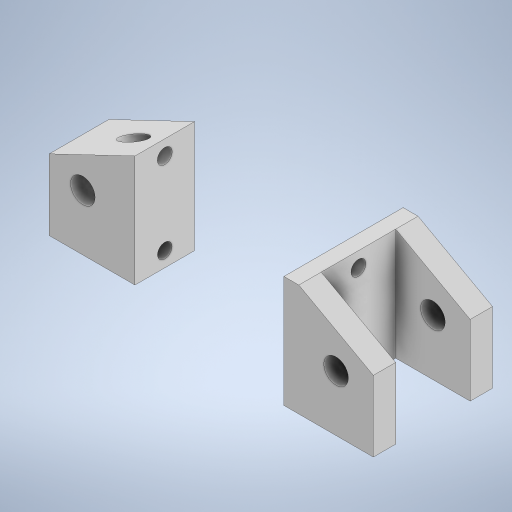
# Autodesk Inventor part: baseFingerLayout
Saved by Autodesk Inventor 2024 (Build 280153000, 153)
## iProperties
Created: 2024-05-29
Part Number: baseFingerLayout
Material: Generic
Document SubType Name: Modeling
Designer: 7008661
Density: 1 g/cm^3
Appearance: Default
Author: 7008661
Autodesk Inventor part; units mm, degrees
ref_plane "YZ Plane" through (0, 0, 0) normal (1, 0, 0) x (0, 1, 0)
ref_plane "XZ Plane" through (0, 0, 0) normal (0, 1, 0) x (-1, 0, 0)
ref_plane "XY Plane" through (0, 0, 0) normal (0, 0, 1) x (1, 0, 0)
sketch "Sketch1" plane through (0, 0, 0) normal (0, 1, 0) x (-1, 0, 0)
  line L0 (-18, -8) -> (18, -8)
  line L1 (18, -8) -> (18, 8)
  line L2 (18, 8) -> (-18, 8)
  line L3 (-18, 8) -> (-18, -8)
  line L4 (-18, -8) -> (18, 8) construction
  line L5 (18, -8) -> (-18, 8) construction
  point P0 (0, 0)
  dimension "d0" = 36
  dimension "d1" = 16
  constraints: 12 end point, 2 midpoint, 2 parallel, 1 horizontal, 1 perpendicular
  measures "d0" distance of L2.end L1.end
  measures "d1" distance of L1.end L0.end
extrude "Extrusion1" add sketch "Sketch1" along normal blind 15
sketch "Sketch2" plane through (18, 0, 8) normal (1, 0, 0) x (0, 0, -1)
  line L0 (16, 15) -> (0, 15) projected
  line L1 (13, 0) -> (3, 0)
  line L2 (3, 0) -> (3, 15)
  line L3 (3, 15) -> (13, 15)
  line L4 (13, 15) -> (13, 0)
  line L5 (13, 0) -> (3, 15) construction
  line L6 (3, 0) -> (13, 15) construction
  point P0 (8, 0)
  point P1 (8, 7.5)
  dimension "d4" = 10
  constraints: 12 end point, 2 midpoint, 2 parallel, 1 horizontal, 1 perpendicular, 1 point on line
  measures "d4" distance of L2.end L3.end
sketch "Sketch3" plane through (-18, 0, 8) normal (0, 0, 1) x (1, 0, 0)
  line L0 (36, 0) -> (36, 15) projected
  line L1 (0, 15) -> (36, 15) projected
  line L2 (36, 0) -> (26, 0)
  line L3 (26, 0) -> (26, 15)
  line L4 (26, 15) -> (36, 15)
  line L5 (36, 15) -> (36, 0)
  circle A0 centre (31, 7.5) radius 1.65
  point P0 (18, 0)
  dimension "d5" = 10
  dimension "d6" = 3.3
  constraints: 8 end point, 2 parallel, 1 centre point, 1 horizontal, 1 perpendicular, 1 point on line
  measures "d5" distance of L3.end L4.end
  measures "d6" diameter of A0
extrude "Extrusion2" cut sketch "Sketch3" against normal blind 21.25 contours A0
chamfer "Chamfer1" distance 10 distance2 5.5 1 edges at (18, 15, 0) measured on face at (17.5, 15, 0)
extrude "Extrusion3" cut sketch "Sketch2" against normal blind 10
sketch "Sketch4" plane through (-18, 0, -8) normal (-1, 0, 0) x (0, 0, 1)
  line L0 (0, 15) -> (16, 15) projected
  line L1 (11.5, 0) -> (4.5, 0)
  line L2 (4.5, 0) -> (4.5, 15)
  line L3 (4.5, 15) -> (11.5, 15)
  line L4 (11.5, 15) -> (11.5, 0)
  line L5 (11.5, 0) -> (4.5, 15) construction
  line L6 (4.5, 0) -> (11.5, 15) construction
  point P0 (8, 0)
  point P1 (8, 7.5)
  dimension "d14" = 7
  constraints: 12 end point, 2 midpoint, 2 parallel, 1 horizontal, 1 perpendicular, 1 point on line
  measures "d14" distance of L2.end L3.end
extrude "Extrusion4" add sketch "Sketch4" along normal blind 11.5
sketch "Sketch5" plane through (-18, 0, 3.5) normal (0, 0, 1) x (1, 0, 0)
  circle A0 centre (-5.75, 7.5) radius 1.65
  point P0 (18, 0)
  dimension "d17" = 3.3
  constraints: 1 centre point
  measures "d17" diameter of A0
extrude "Extrusion5" add sketch "Sketch5" against normal blind 1
chamfer "Chamfer2" distance 6 distance2 11.5 1 edges at (-29.5, 15, 0) measured on face at (-29.5, 14.5, 0)
sketch "Sketch6" plane through (-29.5, 0, -8) normal (-1, 0, 0) x (0, 0, 1)
  point P0 (8, 0)
sketch "Sketch7" plane through (0, 0, 0) normal (0, -1, 0) x (1, 0, 0)
  line L0 (-18, -3.5) -> (-29.5, -3.5) projected
  line L1 (-29.5, 3.5) -> (-18, 3.5) projected
  line L2 (-18, -3.5) -> (-29.5, -3.5)
  line L3 (-29.5, -3.5) -> (-29.5, 3.5)
  line L4 (-29.5, 3.5) -> (-18, 3.5)
  line L5 (-18, 3.5) -> (-18, -3.5)
  point P0 (0, 0)
  constraints: 8 end point, 2 parallel, 1 horizontal, 1 perpendicular
extrude "Extrusion6" add sketch "Sketch7" against normal blind 15
sketch "Sketch8" plane through (-18, 0, -3.5) normal (0, 0, -1) x (-1, 0, 0)
  line L0 (0, 15) -> (11.5, 15) projected
  line L1 (0, 0) -> (11.5, 0) projected
  line L2 (11.5, 15) -> (2.5, 15)
  line L3 (2.5, 15) -> (2.5, 0)
  line L4 (2.5, 0) -> (11.5, 0)
  line L5 (11.5, 0) -> (11.5, 15)
  circle A0 centre (7, 7.5) radius 1.65
  point P0 (-18, 0)
  dimension "d25" = 9
  dimension "d26" = 3.3
  constraints: 8 end point, 2 parallel, 1 centre point, 1 horizontal, 1 perpendicular, 1 point on line
  measures "d25" distance of L4.end L3.end
  measures "d26" diameter of A0
extrude "Extrusion7" cut sketch "Sketch8" along normal mid plane 45.25 contours A0
chamfer "Chamfer3" distance 11.5 distance2 5.5 1 edges at (-29.5, 15, 0) measured on face at (-29, 15, 0)
sketch "Sketch9" plane through (18, 0, -8) normal (0, 0, -1) x (-1, 0, 0)
  point P0 (18, 0)
sketch "Sketch10" plane through (8, 0, 8) normal (1, 0, 0) x (0, 0, -1)
  line L0 (4.5, 15) -> (11.5, 15) projected
  circle A0 centre (8, 13) radius 1
  circle A1 centre (8, 2) radius 0.975
  point P0 (8, 0)
  dimension "d32" = 2
  constraints: 2 centre point
  measures "d32" diameter of A0
extrude "Extrusion8" cut sketch "Sketch10" against normal blind 65.75
sketch "Sketch11" plane through (-29.5, 0, 3.5) normal (0, 0, 1) x (1, 0, 0)
  line L0 (0, 0) -> (0, 9.5) projected
  line L1 (37.5, 15) -> (11.5, 15) projected
  line L2 (0, 9.5) -> (11.5, 15)
  line L3 (47.5, 0) -> (11.5, 0) projected
  line L4 (11.5, 15) -> (11.5, 0)
  line L5 (11.5, 0) -> (0, 0)
  line L6 (0, 0) -> (0, 9.5)
  point P0 (29.5, 0)
  constraints: 8 end point, 3 perpendicular
extrude "Extrusion9" add sketch "Sketch11" along normal blind 0.5
sketch "Sketch12" plane through (-18, 0, -3.5) normal (0, 0, -1) x (-1, 0, 0)
  circle A0 centre (7, 7.5) radius 1.65 projected
  circle A1 centre (7, 7.5) radius 1.65
  point P0 (-18, 0)
  constraints: 1 centre point, 1 coincident
extrude "Extrusion10" cut sketch "Sketch12" against normal blind 9
sketch "Sketch13" plane through (-18, 0, -3.5) normal (0, 0, -1) x (-1, 0, 0)
  point P0 (-18, 0)
sketch "Sketch14" plane through (-18, 0, -3.5) normal (0, 0, -1) x (-1, 0, 0)
  line L0 (0, 0) -> (0, 15) projected
  line L1 (0, 0) -> (0, 15)
  line L2 (11.5, 9.5) -> (11.5, 0) projected
  line L3 (0, 15) -> (11.5, 9.5)
  line L4 (11.5, 9.5) -> (11.5, 0)
  line L5 (11.5, 0) -> (0, 0) projected
  line L6 (11.5, 0) -> (0, 0)
  point P0 (-18, 0)
  constraints: 8 end point, 2 collinear, 1 parallel
extrude "Extrusion11" add sketch "Sketch14" along normal blind 0.5
sketch "Sketch15" plane through (-29.5, 0, 4) normal (0, 0, 1) x (1, 0, 0)
  circle A0 centre (4.5, 7.5) radius 1.65 projected
  circle A1 centre (4.5, 7.5) radius 1.65
  point P0 (29.5, 0)
  constraints: 1 centre point, 1 coincident
extrude "Extrusion12" cut sketch "Sketch15" against normal blind 13
sketch "Sketch16" plane through (0, 15, 0) normal (0, 1, 0) x (1, 0, 0)
  line L0 (-18, -4) -> (-18, -8) projected
  line L1 (8, 8) -> (-18, 8) projected
  line L2 (-18, -8) -> (6, -8)
  line L3 (6, -8) -> (6, 8)
  line L4 (6, 8) -> (-18, 8)
  line L5 (-18, 8) -> (-18, -8)
  point P0 (0, 0)
  dimension "d43" = 24
  constraints: 8 end point, 2 parallel, 1 horizontal, 1 perpendicular, 1 point on line
  measures "d43" distance of L4.end L3.end
extrude "Extrusion13" cut sketch "Sketch16" against normal blind 21
ref_plane "Work Plane1" through (-6.25, 15, -8) normal (-1, 0, 0) x (0, 0, 1)
split body "Split1" result two bodies by plane through (-6.25, 15, -8) normal (-1, 0, 0) first body at (-19.7833, 7.5, -3.5)
body "Solid2"
body "Solid3"
